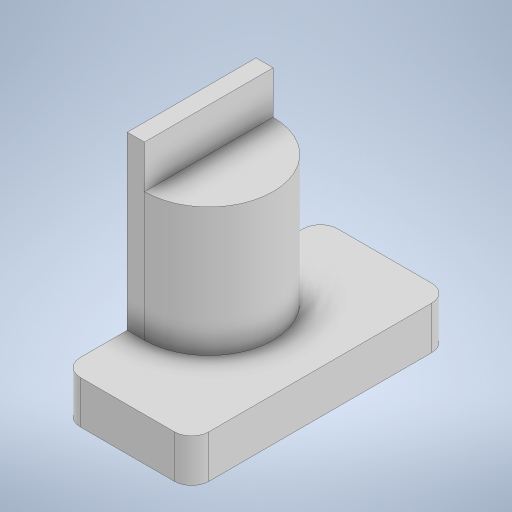
# Autodesk Inventor part: 孔1
Saved by Autodesk Inventor 2024.2 (Build 282272000, 272)
## iProperties
Created: 2024-03-28
Part Number: 孔1
Material: 一般
Document SubType Name: Modeling
Designer: User
Density: 1 g/cm^3
Appearance: 預設
Author: User
Autodesk Inventor part; units mm, degrees
ref_plane "YZ Plane" through (0, 0, 0) normal (1, 0, 0) x (0, 1, 0)
ref_plane "XZ Plane" through (0, 0, 0) normal (0, 1, 0) x (-1, 0, 0)
ref_plane "XY Plane" through (0, 0, 0) normal (0, 0, 1) x (1, 0, 0)
sketch "草圖1" plane through (0, 0, 0) normal (0, 1, 0) x (-1, 0, 0)
  line L0 (0, 0) -> (-15, 0)
  line L1 (-15, 0) -> (-15, -30)
  line L2 (-15, -30) -> (0, -30)
  line L3 (0, -30) -> (0, 0)
  dimension "d0" = 15
  dimension "d1" = 30
  constraints: 8 end point, 2 parallel, 1 horizontal, 1 perpendicular
  measures "d0" distance of L2.end L1.end
  measures "d1" distance of L1.end L0.end
extrude "擠出1" add sketch "草圖1" along normal blind 5
fillet "圓角1" radius 2 4 edges at (15, 2.5, 0) (15, 2.5, -30) (0, 2.5, 0) (0, 2.5, -30)
sketch "草圖2" plane through (0, 5, 0) normal (0, 1, 0) x (1, 0, 0)
  line L0 (13, 30) -> (2, 30) projected
  line L1 (0, 28) -> (0, 2) projected
  line L2 (2, 30) -> (2, 15)
  arc A0 (2, 7.5) -> (2, 22.5) centre (2, 15) ccw
  line L3 (2, 15) -> (2, 7.5)
  line L4 (2, 15) -> (2, 22.5)
  line L5 (2, 22.5) -> (0, 22.5)
  line L6 (2, 7.5) -> (0, 7.5)
  line L7 (0, 22.5) -> (0, 7.5)
  point P0 (0, 0)
  dimension "d8" = 15
  dimension "d9" = 15
  constraints: 12 end point, 2 point on circle, 2 point on line, 2 vertical, 1 centre point, 1 coincident, 1 horizontal, 1 midpoint, 1 perpendicular
  measures "d8" distance of L0.end L2.end
  measures "d9" diameter of A0
extrude "擠出3" add sketch "草圖2" along normal blind 15 contours A0 L3 L2
extrude "擠出4" add sketch "草圖2" along normal blind 20 contours L5 L2 L3 L6 L1
